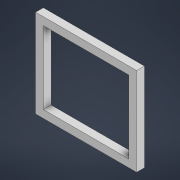
# Autodesk Inventor part: End-Effector
Saved by Autodesk Inventor 2022 (Build 260153000, 153)
## iProperties
Created: 2023-04-20
Part Number: End-Effector
Material: Generic
Document SubType Name: Modeling
Designer: Karl
Density: 1 g/cm^3
Appearance: Default
Author: Karl
Autodesk Inventor part; units mm, degrees
ref_plane "YZ Plane" through (0, 0, 0) normal (1, 0, 0) x (0, 1, 0)
ref_plane "XZ Plane" through (0, 0, 0) normal (0, 1, 0) x (-1, 0, 0)
ref_plane "XY Plane" through (0, 0, 0) normal (0, 0, 1) x (1, 0, 0)
sketch "Sketch3" plane through (0, 0, 0) normal (0, 0, 1) x (1, 0, 0)
  line L0 (0, 0) -> (-55.38, 0)
  line L1 (-55.38, 0) -> (-55.38, 47.03)
  line L2 (-55.38, 47.03) -> (0, 47.03)
  line L3 (0, 47.03) -> (0, 0)
  line L4 (5, -5) -> (5, 52.03)
  line L5 (5, 52.03) -> (-60.38, 52.03)
  line L6 (5, -5) -> (-60.38, -5)
  line L7 (-60.38, -5) -> (-60.38, 52.03)
  dimension "d26" = 47.03
  dimension "d27" = 55.38
  constraints: 16 end point, 3 perpendicular, 2 horizontal, 2 parallel, 1 vertical
  measures "d26" distance of L2.end L0.start
  measures "d27" distance of L0.start L0.end
extrude "Extrusion10" add sketch "Sketch3" along normal blind 5
body "Solid3"
